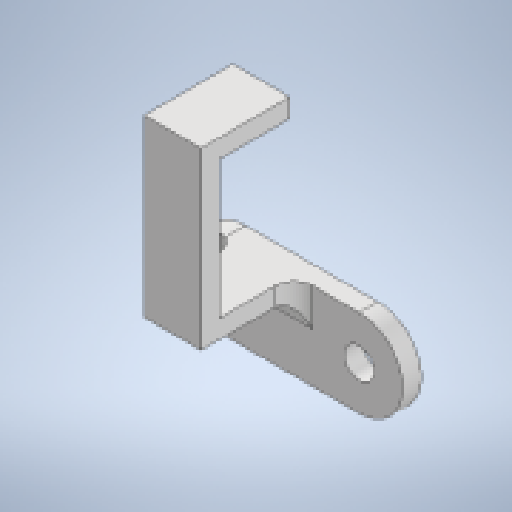
# Autodesk Inventor part: j3 endstop blocker
Saved by Autodesk Inventor 2025 (Build 290162000, 162)
## iProperties
Created: 2025-08-04
Part Number: j3 endstop blocker
Material: 一般
Document SubType Name: Modeling
Designer: gavin
Density: 1 g/cm^3
Appearance: 預設
Author: gavin
## iProperties of the stored document j3 endstop blocker_3D 列印.ipt
Created: 2025-08-04
Part Number: j3 endstop blocker_3D 列印
Material: 一般
Document SubType Name: Modeling
Designer: gavin
Density: 1 g/cm^3
Appearance: 預設
Author: gavin
Autodesk Inventor part; units mm, degrees
ref_plane "工作平面1" through (0, 0, 0) normal (0, 0, 1) x (1, 0, 0)
sketch "草圖1" plane through (0, 0, 0) normal (0, 0, 1) x (1, 0, 0)
  circle A0 centre (-7.075, 38.25) radius 2.165 projected
  circle A1 centre (7.075, 38.25) radius 2.165 projected
  arc A2 (-15.075, -26.25) -> (-13.075, -28.25) centre (-13.075, -26.25) ccw projected
  line L0 (-13.075, -28.25) -> (13.075, -28.25) projected
  arc A3 (13.075, -28.25) -> (15.075, -26.25) centre (13.075, -26.25) ccw projected
  line L1 (15.075, -26.25) -> (15.075, 43.25) construction
  line L2 (-15.075, 43.25) -> (15.075, 43.25) construction
  line L3 (-15.075, 43.25) -> (-15.075, -26.25) construction
  line L4 (-10.075, 23.25) -> (10.075, 23.25) projected
  line L5 (10.075, 23.25) -> (10.075, 3.1) projected
  line L6 (10.075, 3.1) -> (-10.075, 3.1) projected
  line L7 (-10.075, 3.1) -> (-10.075, 23.25) projected
  line L8 (-10.075, -3.1) -> (10.075, -3.1) projected
  line L9 (10.075, -3.1) -> (10.075, -23.25) projected
  line L10 (10.075, -23.25) -> (-10.075, -23.25) projected
  line L11 (-10.075, -23.25) -> (-10.075, -3.1) projected
  arc A4 (7.075, 33.585) -> (7.075, 42.915) centre (7.075, 38.25) ccw
  arc A5 (-7.075, 42.915) -> (-7.075, 33.585) centre (-7.075, 38.25) ccw
  line L12 (7.075, 33.585) -> (-7.075, 33.585)
  line L13 (7.075, 42.915) -> (-7.075, 42.915)
  circle A6 centre (7.075, 38.25) radius 1.6
  circle A7 centre (-7.075, 38.25) radius 1.6
  point P0 (0, 0)
  dimension "d0" = 2.5
  dimension "d1" = 2.5
  dimension "d20" = 3.2
  dimension "d21" = 3.2
  constraints: 4 centre point, 4 end point, 4 point on circle, 2 coincident, 1 horizontal, 1 tangent
  measures "d0" radial gap between concentric circles of A1 A4
  measures "d1" radial gap between concentric circles of A0 A5
  measures "d20" diameter of A6
  measures "d21" diameter of A7
extrude "擠出1" add sketch "草圖1" along normal blind 2 contours A0 | A1 | L12 A5 L13 A4
ref_plane "工作平面3" through (-5.8702, 48.2125, -2.9174) normal (-0.9999955, 0, 0.0030077) x (0.0030077, 0, 0.9999955)
ref_plane "工作平面4" through (0.1, 52.2125, 8.4448) normal (1, 0, 0) x (0, 1, 0)
sketch "草圖3" plane through (0.1, 52.2125, 8.4448) normal (1, 0, 0) x (0, 1, 0)
  line L0 (-18.6275, -8.4448) -> (-9.2975, -8.4448) projected
  line L1 (-9.2975, -8.4448) -> (-9.2975, -6.4448) projected
  line L2 (-18.6275, -6.4448) -> (-9.2975, -6.4448) projected
  line L3 (-18.6275, -8.4448) -> (-18.6275, -6.4448) projected
  line L4 (4, -7.96) -> (4, 0) projected
  line L5 (4, 0) -> (0, 0) projected
  line L6 (0, 0) -> (0, -9.8) projected
  line L7 (12.94, -9.8) -> (0, -9.8) projected
  line L8 (12.94, -9.8) -> (12.94, 0) projected
  line L9 (12.94, 0) -> (8.94, 0) projected
  line L10 (8.94, 0) -> (8.94, -7.96) projected
  line L11 (8.94, -7.96) -> (4, -7.96) projected
  line L12 (-9.2975, -6.4448) -> (-9.2975, 1.5)
  line L13 (-9.2975, 1.5) -> (5.4231, 1.5)
  line L14 (5.4231, 1.5) -> (5.4231, -6)
  line L15 (5.4231, -6) -> (7.4231, -6)
  line L16 (7.4231, -6) -> (7.4231, 3.5)
  line L17 (7.4231, 3.5) -> (-11.2975, 3.5)
  line L18 (-11.2975, 3.5) -> (-11.2975, -6.4448)
  point P0 (-52.2125, -8.4448)
  point P1 (-9.2975, 3.5)
  dimension "d12" = 2
  dimension "d13" = 2
  dimension "d14" = 2
  dimension "d15" = 1.5
  dimension "d16" = 7.5
  constraints: 14 end point, 6 perpendicular, 1 point on line, 1 vertical
  measures "d12" distance of L14.end L15.end
  measures "d13" distance between parallel lines of L17 L13
  measures "d14" distance between parallel lines of L18 L12
  measures "d15" distance from line of L13 L5.end
  measures "d16" distance of L13.end L14.end
extrude "擠出3" add sketch "草圖3" against normal blind 6.1 contours L2 L18 L17 L16 L15 L14 L13 L12
fillet "圓角1" radius 2 3 edges at (0.1, 41.915, 2) (-2.95, 40.915, 2) (-6, 41.915, 2)
